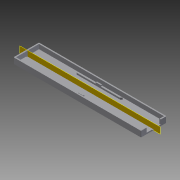
# Autodesk Inventor part: Base
Saved by Autodesk Inventor 2011 (Build 150239000, 239)
## iProperties
Created: 2014-08-04
Part Number: Base
Document SubType Name: Modeling
Designer: amatiasq
Density: 1 g/cm^3
Author: amatiasq
Autodesk Inventor part; units mm, degrees
ref_plane "YZ Plane" through (0, 0, 0) normal (1, 0, 0) x (0, 1, 0)
ref_plane "XZ Plane" through (0, 0, 0) normal (0, 1, 0) x (-1, 0, 0)
ref_plane "XY Plane" through (0, 0, 0) normal (0, 0, 1) x (1, 0, 0)
sketch "Boceto1" plane through (0, 0, 0) normal (0, 0, 1) x (1, 0, 0)
  line L0 (0, 0) -> (200, 0)
  line L1 (200, 0) -> (200, 40)
  line L2 (200, 40) -> (0, 40)
  line L3 (0, 40) -> (0, 0)
  dimension "d0" = 200
  dimension "d1" = 40
  constraints: 8 end point, 2 parallel, 1 horizontal, 1 perpendicular
  measures "d0" distance of L2.end L1.end
  measures "d1" distance of L1.end L0.end
extrude "Base" add sketch "Boceto1" along normal blind 2
sketch "Boceto2" plane through (0, 0, 2) normal (0, 0, 1) x (1, 0, 0)
  line L0 (200, 40) -> (200, 0) projected
  line L1 (200, 22) -> (2, 22)
  line L2 (2, 22) -> (2, 18)
  line L3 (2, 18) -> (200, 18)
  line L4 (200, 18) -> (200, 22)
  point P0 (0, 40)
  point P1 (200, 20)
  dimension "d4" = 4
  dimension "d5" = 2
  constraints: 8 end point, 2 midpoint, 2 parallel, 1 horizontal, 1 perpendicular
  measures "d4" distance of L2.end L1.end
  measures "d5" horizontal distance of point (0, 40) L1.end
extrude "Canal" cut sketch "Boceto2" against normal blind 1
sketch "Boceto3" plane through (0, 0, 2) normal (0, 0, 1) x (1, 0, 0)
  line L0 (2, 22) -> (200, 22) projected
  line L1 (200, 40) -> (200, 22) projected
  line L2 (0, 40) -> (200, 40) projected
  line L3 (0, 0) -> (0, 40) projected
  line L4 (200, 0) -> (0, 0) projected
  line L5 (200, 18) -> (200, 0) projected
  line L6 (200, 18) -> (2, 18) projected
  line L7 (198, 38) -> (2, 38)
  line L8 (2, 38) -> (2, 2)
  line L9 (2, 2) -> (198, 2)
  line L10 (198, 2) -> (198, 9)
  line L11 (198, 9) -> (200, 9)
  line L12 (198, 38) -> (198, 31)
  line L13 (198, 31) -> (200, 31)
  dimension "d8" = 2
  dimension "d9" = 2
  dimension "d10" = 2
  dimension "d11" = 2
  dimension "d12" = 2
  dimension "d33" = 7
  dimension "d34" = 7
  constraints: 14 end point, 3 parallel, 3 perpendicular, 2 midpoint
  measures "d8" horizontal distance of L1.start L7.start
  measures "d9" horizontal distance of L2.start L7.end
  measures "d10" horizontal distance of L3.start L8.end
  measures "d11" horizontal distance of L2.start L7.end
  measures "d12" horizontal distance of L4.start L9.end
  measures "d33" distance of L9.end L10.end
  measures "d34" distance of L7.start L12.end
extrude "Paredes" add sketch "Boceto3" along normal blind 7 contours L8 L9 L10 L11 L5 L4 L3 L2 L1 L13 L12 L7
sketch "Boceto4" plane through (0, 0, 2) normal (0, 0, 1) x (1, 0, 0)
  point P0 (0, 0)
  point P1 (49, 4)
  point P2 (151, 4)
hole "Hole1" at (49, 4, 2) at (151, 4, 2) direction (0, 0, -1) diameter 1 end through all
fillet "Empalme1" radius 1 4 edges at (200, 40, 4.5) (200, 0, 4.5) (0, 40, 4.5) (0, 0, 4.5)
sketch "Boceto5" plane through (0, 0, 2) normal (0, 0, 1) x (1, 0, 0)
  line L0 (2, 38) -> (2, 22) projected
  line L1 (198, 22) -> (198, 38) projected
  line L2 (198, 38) -> (2, 38) projected
  line L3 (136, 35) -> (64, 35)
  line L4 (64, 35) -> (66, 33)
  line L5 (66, 33) -> (134, 33)
  line L6 (134, 33) -> (136, 35)
  point P0 (0, 0)
  dimension "d23" = 2
  dimension "d24" = 2
  dimension "d25" = 3
  dimension "d26" = 62
  dimension "d27" = 62
  constraints: 8 end point, 2 parallel, 1 perpendicular
  measures "d23" horizontal distance of L3.start L5.end
  measures "d24" horizontal distance of L3.start L5.end
  measures "d25" distance from line of L2 L3.end
  measures "d26" distance from line of L0 L3.end
  measures "d27" distance from line of L1 L3.start
extrude "Extrusión4" add sketch "Boceto5" along normal blind 2.5
sketch "Boceto6" plane through (0, 0, 4.5) normal (0, 0, 1) x (1, 0, 0)
  line L0 (64, 35) -> (136, 35) projected
  line L1 (134, 33) -> (66, 33) projected
  line L2 (96, 35) -> (104, 35)
  line L3 (104, 35) -> (104, 33)
  line L4 (104, 33) -> (96, 33)
  line L5 (96, 33) -> (96, 35)
  point P0 (0, 0)
  point P1 (100, 35)
  dimension "d30" = 8
  constraints: 8 end point, 2 midpoint, 2 parallel, 2 point on line, 1 horizontal, 1 perpendicular
  measures "d30" distance of L2.end L2.start
extrude "Extrusión5" add sketch "Boceto6" along normal blind 2
ref_plane "Mitad" through (1, 20, 0) normal (0, 1, 0) x (1, 0, 0)
mirror "Simetría1" about plane through (1, 20, 0) normal (0, 1, 0) of "Extrusión4", "Extrusión5"
